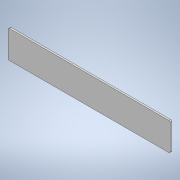
# Autodesk Inventor part: lamina1
Saved by Autodesk Inventor 2021 (Build 250183000, 183)
## iProperties
Created: 2022-05-07
Part Number: lamina1
Material: Genérico
Document SubType Name: Modeling
Designer: luzve
Density: 1 g/cm^3
Appearance: Valor por defecto
Author: luzve
Autodesk Inventor part; units mm, degrees
ref_plane "YZ Plane" through (0, 0, 0) normal (1, 0, 0) x (0, 1, 0)
ref_plane "XZ Plane" through (0, 0, 0) normal (0, 1, 0) x (-1, 0, 0)
ref_plane "XY Plane" through (0, 0, 0) normal (0, 0, 1) x (1, 0, 0)
sketch "Boceto1" plane through (0, 0, 0) normal (0, 0, 1) x (1, 0, 0)
  line L0 (0, 0) -> (290, 0)
  line L1 (290, 0) -> (290, 50)
  line L2 (290, 50) -> (0, 50)
  line L3 (0, 50) -> (0, 0)
  dimension "d0" = 290
  dimension "d1" = 50
  constraints: 8 end point, 2 parallel, 1 horizontal, 1 perpendicular
  measures "d0" distance of L2.end L1.end
  measures "d1" distance of L1.end L0.end
extrude "Extrusión1" add sketch "Boceto1" along normal blind 3
fillet "Empalme1" radius 2 4 edges at (290, 50, 1.5) (290, 0, 1.5) (0, 0, 1.5) (0, 50, 1.5)
